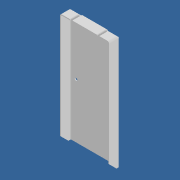
# Autodesk Inventor part: Display_Angle
Saved by Autodesk Inventor 2020 (Build 240168000, 168)
## iProperties
Created: 2021-04-28
Part Number: Display_Angle
Material: 一般
Document SubType Name: Sheet Metal
Designer: ken113
Density: 1 g/cm^3
Sheet Metal Rule: Default_mm
Appearance: 既定
Author: ken113
Autodesk Inventor part; units mm, degrees
ref_plane "YZ Plane" through (0, 0, 0) normal (1, 0, 0) x (0, 1, 0)
ref_plane "XZ Plane" through (0, 0, 0) normal (0, 1, 0) x (-1, 0, 0)
ref_plane "XY Plane" through (0, 0, 0) normal (0, 0, 1) x (1, 0, 0)
sketch "スケッチ1" plane through (0, 0, 0) normal (0, 0, 1) x (1, 0, 0)
  line L0 (-50, 0) -> (50, 0)
  line L1 (50, 0) -> (50, -227)
  line L2 (50, -227) -> (-50, -227)
  line L3 (-50, -227) -> (-50, 0)
  point P0 (0, 0)
  dimension "d0" = 100
  dimension "d1" = 50
  dimension "d2" = 227
  measures "d0" distance of L1.end L2.end
  measures "d1" distance from line of point (0, 0) L3
  measures "d2" distance of L0.end L1.end
extrude "プレート1" add sketch "スケッチ1" along normal blind 2
sketch "スケッチ2" plane through (48, 0, 0) normal (1, 0, 0) x (0, 1, 0)
  line L0 (-227, 0) -> (0, 0)
  line L1 (0, 0) -> (0, 22)
  line L2 (0, 22) -> (-227, 22)
  line L3 (-227, 22) -> (-227, 0)
  constraints: 6 end point, 1 horizontal, 1 perpendicular, 1 vertical
edge flange "フランジ1" height 22 angle 90 thickness 2 bend radius 2 thickness toward (1, 0, 0) relief straight relief width 2 relief depth 1 corner gap 2 corner form 0 edges at (50, -113.5, 2) (-50, -113.5, 2) wall of the first edge with corners at (48, -227, 0) (48, 0, 0) (48, 0, 22) (48, -227, 22)
bend "曲げ1"
corner "コーナー1"
sketch "スケッチ6" plane through (-46, 2, 22) normal (0, 1, 0) x (-1, 0, 0)
  line L0 (0, -18) -> (0, 0)
  line L1 (0, 0) -> (-16, 0)
  line L2 (-16, 0) -> (-16, -18)
  line L3 (-16, -18) -> (0, -18)
  constraints: 6 end point, 1 horizontal, 1 perpendicular, 1 vertical
edge flange "フランジ5" height 20 angle 90 thickness 2 bend radius 2 thickness toward (0, 1, 0) relief straight relief width 2 relief depth 1 corner gap 2 corner form 0 edges at (-48, 0, 13) (48, 0, 13) wall of the first edge with corners at (-46, 2, 4) (-46, 2, 22) (-30, 2, 22) (-30, 2, 4)
bend "曲げ5"
corner "コーナー5"
sketch "スケッチ7" plane through (0, 0, 2) normal (0, 0, 1) x (1, 0, 0)
  line L0 (-25, 0) -> (25, 0)
  line L1 (25, 0) -> (25, 2)
  line L2 (25, 2) -> (-25, 2)
  line L3 (-25, 2) -> (-25, 0)
  line L4 (-30, 2) -> (-30, 4) projected
  line L5 (30, 2) -> (30, 4) projected
  point P0 (0, 0)
  dimension "d55" = 2
  dimension "d56" = 5
  dimension "d57" = 5
  constraints: 8 end point, 2 parallel, 1 horizontal, 1 perpendicular
  measures "d55" distance of L0.end L1.end
  measures "d56" distance between parallel lines of L4 L3
  measures "d57" distance between parallel lines of L5 L1
extrude "押し出し1" add sketch "スケッチ7" against normal up to surface (2 mm away)
sketch "スケッチ8" plane through (-25, 2, 2) normal (0, 1, 0) x (-1, 0, 0)
  line L0 (-50, 0) -> (0, 0)
  line L1 (0, 0) -> (0, 20)
  line L2 (0, 20) -> (-50, 20)
  line L3 (-50, 20) -> (-50, 0)
  constraints: 6 end point, 1 horizontal, 1 perpendicular, 1 vertical
edge flange "フランジ6" height 20 angle 90 thickness 2 bend radius 2 thickness toward (0, 1, 0) relief straight relief width 2 relief depth 1 edges at (0, 2, 2) wall of the first edge with corners at (25, 2, 2) (-25, 2, 2) (-25, 2, 22) (25, 2, 22)
bend "曲げ6"
corner "コーナー6"
sketch "スケッチ9" plane through (0, 0, 2) normal (0, 0, 1) x (1, 0, 0)
  line L0 (25, 4) -> (-25, 4) projected
  point P0 (0, 0)
  point P1 (-37.5, -116)
  point P2 (37.5, -116)
  dimension "d71" = 75
  dimension "d72" = 37.5
  dimension "d73" = 120
  constraints: 1 horizontal alignment
  measures "d71" distance of point (37.5, -116) point (-37.5, -116)
  measures "d72" horizontal distance of point (0, 0) point (-37.5, -116)
  measures "d73" distance from line of point (37.5, -116) L0
hole "穴1" at (-37.5, -116, 2) at (37.5, -116, 2) direction (0, 0, -1) diameter 5.2 depth 2 tip angle 118
chamfer "面取り1" distance 15 angle 45 2 edges at (-49, -227, 22) (49, -227, 22)
equation "\"d72\" = 0.5 * d71"
equation "\"d79\" = Thickness"
equation "\"d3\" = Thickness"
equation "\"d4\" = BendReliefWidth"
equation "\"d5\" = BendReliefDepth"
equation "\"d6\" = MinimumRemnant"
equation "\"d7\" = TransitionRadius"
equation "\"d10\" = BendRadius"
equation "\"d11\" = CornerReliefSize"
equation "\"d12\" = GapSize"
equation "\"d13\" = JacobiRadiusSize"
equation "\"d45\" = BendReliefWidth"
equation "\"d46\" = BendReliefDepth"
equation "\"d47\" = MinimumRemnant"
equation "\"d48\" = TransitionRadius"
equation "\"d51\" = BendRadius"
equation "\"d52\" = CornerReliefSize"
equation "\"d53\" = GapSize"
equation "\"d54\" = JacobiRadiusSize"
equation "\"d60\" = BendReliefWidth"
equation "\"d61\" = BendReliefDepth"
equation "\"d62\" = MinimumRemnant"
equation "\"d63\" = TransitionRadius"
equation "\"d66\" = BendRadius"
equation "\"d68\" = CornerReliefSize"
equation "\"d69\" = GapSize"
equation "\"d70\" = JacobiRadiusSize"
equation "\"d1\" = 0.5 * d0"
equation "\"BendRadius\" = Thickness"
equation "\"BendReliefWidth\" = Thickness"
equation "\"BendReliefDepth\" = 0.5 * Thickness"
equation "\"CornerReliefSize\" = 4 * Thickness"
equation "\"MinimumRemnant\" = 2 * Thickness"
equation "\"TransitionRadius\" = BendRadius"
equation "\"JacobiRadiusSize\" = BendRadius"
equation "\"GapSize\" = Thickness"
equation "\"Thickness\" = 2"
